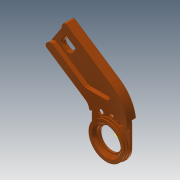
# Autodesk Inventor part: J009523
Saved by Autodesk Inventor 2020 (Build 240168000, 168)
## iProperties
RuleStatus: InUse
AfterDocSave0: file://Part Number Cleaner
Created: 2014-10-29
Material: TITANIUM, 6AL-4V, ANNEALED
Vendor: HHMI: JRC - JET
Document SubType Name: Modeling
Designer: arnoldj
Density: 4.43 g/cm^3
Description: MBS INLINE RING TAB THIN
Mass: 2.07661 g
Surface Area: 8.87594 cm^2
Volume: 0.468761 cm^3
Project: COMMON
Appearance: Smooth - Light Orange
Sheet Metal Rule: Default
Part Number: J009523
DESIGN DEPARTMENT: HHMI: JRC - ID&F
SPECIAL FINISH: NONE
LAB/DEPT: COMMON
REQUESTING SCIENTIST: COMMON
SURFACE ROUGHNESS: 63 Ra
Thickness: 0.100 in
ALTERED ITEM PART NUMBER: N/A
ALTERED ITEM VENDOR: N/A
ALTERED ITEM DESCRIPTION: N/A
Revision Number: -
Autodesk Inventor part; units mm, degrees
ref_plane "YZ Plane" through (0, 0, 0) normal (1, 0, 0) x (0, 1, 0)
sketch "Sketch1" plane through (0, 0, 0) normal (0, 0, 1) x (1, 0, 0)
  line L0 (-5.334, -5) -> (-5.334, 6.0312)
  line L1 (-5.334, 6.0312) -> (-5.334, -2.6352) construction
  line L2 (-5.334, 6.0312) -> (-17.9557, 14.3853)
  line L3 (-17.9557, 14.3853) -> (-12.4181, 22.7517)
  line L4 (-12.4181, 22.7517) -> (5.334, 11.0019)
  line L5 (-17.9557, 14.3853) -> (-30.248, 14.3853) construction
  line L6 (-15.1869, 18.5685) -> (0, 8.5166) construction
  line L7 (-12.1504, 14.2743) -> (-10.0476, 17.4514)
  line L8 (-10.0476, 17.4514) -> (-12.7163, 19.2178)
  line L9 (-12.7163, 19.2178) -> (-14.8192, 16.0407)
  line L10 (-14.8192, 16.0407) -> (-12.1504, 14.2743)
  line L11 (-12.1504, 14.2743) -> (-12.7163, 19.2178) construction
  line L12 (-10.0476, 17.4514) -> (-14.8192, 16.0407) construction
  circle A0 centre (0, 0) radius 3.5 construction
  line L13 (5.334, -5) -> (5.334, 11.0019)
  line L14 (0, 29.0086) -> (0, -14.7897) projected
  line L15 (-38.8526, 0) -> (21.3792, 0) projected
  circle A1 centre (0, 0) radius 3.5
  line L16 (-5.334, -5) -> (5.334, -5)
  point P0 (0, 0)
  point P1 (-2.611, 1.214)
  point P2 (-12.4334, 16.746)
  dimension "d161" = 123.5
  dimension "d162" = 10.033
  dimension "d177" = 146.5
  dimension "d221" = 3.302
  dimension "d232" = 3.2004
  dimension "d233" = 3.81
  dimension "d262" = 7
  dimension "d267" = 0
  dimension "d271" = 16.746
  dimension "d273" = 5.334
  dimension "d274" = 1.834
  dimension "d275" = 5.334
  dimension "d320" = 0
  dimension "d321" = 5
  dimension "d430" = 12.4334
  constraints: 30 end point, 4 coincident, 4 parallel, 4 point on line, 3 midpoint, 3 perpendicular, 3 vertical, 2 centre point, 2 horizontal, 1 concentric
  measures "d161" angle of L2 L0
  measures "d162" distance of L2.end L3.end
  measures "d177" angle of L2 L5
  measures "d221" distance from line of point (-12.433, 16.746) L3
  measures "d232" distance of L7.end L8.end
  measures "d233" distance of L7.start L7.end
  measures "d262" diameter of A0
  measures "d267" distance from line of L15 point (0, 0)
  measures "d271" vertical distance of point (-12.433, 16.746) A1.centre
  measures "d273" distance from line of A0.centre L0
  measures "d274" distance edge to line of A0 L0
  measures "d275" distance from line of A0.centre L13
  measures "d320" distance from line of L14 A0.centre
  measures "d321" distance from line of A0.centre L16
  measures "d430" distance from line of point (-12.433, 16.746) L14
extrude "Plate1" add sketch "Sketch1" along normal blind 2.54 contours L0 L15 A1 L14 L16 | L0 L2 L3 L4 L14 A1 L15 | L14 A1 L15 L13 L16 | L14 L4 L13 L15 A1 | L10 L9 L8 L7
ref_plane "Work Plane1" through (0, 10.16, 0) normal (0, 1, 0) x (-1, 0, 0)
sketch "Sketch7" plane through (0, 0, 0) normal (0, 0, 1) x (1, 0, 0)
  circle A0 centre (0, 6.0325) radius 0.8255
  circle A1 centre (-2.921, 5.1689) radius 0.8255
  circle A2 centre (2.921, 5.1689) radius 0.8255
  line L0 (0, 23.2371) -> (0, -13.8278) construction
  circle A3 centre (-2.1082, 6.9916) radius 0.8255
  circle A4 centre (2.1082, 6.9916) radius 0.8255
  line L1 (-5.334, -5) -> (-5.334, 6.0312) projected
  line L2 (-22.6717, 0) -> (18.6824, 0) projected
  circle A5 centre (0, 0) radius 3.5 projected
  circle A6 centre (0, 0) radius 6.0325 construction
  circle A7 centre (0, 0) radius 7.3025 construction
  dimension "d343" = 12.065
  dimension "d61" = 1.651
  dimension "d344" = 14.605
  dimension "d345" = 2.921
  dimension "d346" = 2.921
  dimension "d347" = 2.1082
  dimension "d348" = 2.1082
  constraints: 6 centre point, 5 coincident, 4 equal radius, 2 point on circle, 1 vertical alignment, 2 other
  measures "d61" diameter of A0
  measures "d344" diameter of A7
  measures "d345" horizontal distance of A0.centre point (2.921, 5.169)
  measures "d346" horizontal distance of point (-2.921, 5.169) A0.centre
  measures "d347" distance from line of L0 point (2.108, 6.992)
  measures "d348" distance from line of L0 A3.centre
hole "Hole2" at (-2.921, 5.1689, 0) at (2.921, 5.1689, 0) at (0, 6.0325, 0) direction (0, 0, 1) diameter 1.651 depth 2.54 tip angle 118
ref_plane "Work Plane3" through (0, 0, 1.143) normal (0, 0, 1) x (1, 0, 0)
sketch "Sketch9" plane through (0, 0, 0) normal (0, 0, 1) x (1, 0, 0)
  point P0 (0, 0)
sketch "Sketch10" plane through (0, 0, 0) normal (0, 0, 1) x (1, 0, 0)
  circle A0 centre (2.6461, -1.2506) radius 3.5
  point P0 (0, 0)
  dimension "d150" = 7
  constraints: 1 centre point
  measures "d150" diameter of A0
sketch "Sketch3" plane through (0, 0, 2.54) normal (0, 0, 1) x (1, 0, 0)
  line L0 (-16.764, 14.16) -> (4.445, 14.16)
  line L1 (-4.445, 6.16) -> (-16.764, 6.16)
  line L2 (-6.35, 14.16) -> (-6.35, 6.16)
  line L3 (0, 17.9421) -> (0, -8.5328)
  line L4 (12.7747, 8.2785) -> (4.445, 8.2785)
  point P0 (0, 0)
  point P1 (-5.2531, 14.0148)
  point P2 (4.445, 14.16)
  dimension "d15" = 6.35
  constraints: 8 end point, 1 perpendicular, 1 point on line, 4 other
  measures "d15" distance between parallel lines of L3 L2
sketch "Sketch15" plane through (0, 0, 0) normal (0, 0, 1) x (1, 0, 0)
  point P0 (0, 0)
extrude "Extrusion7" cut sketch "Sketch1" along normal up to next contours L10 L9 L8 L7
fillet "Fillet19" radius 1.27 4 edges at (-10.0476, 17.4514, 1.27) (-12.1504, 14.2743, 1.27) (-14.8192, 16.0407, 1.27) (-12.7163, 19.2178, 1.27)
sketch "Sketch20" plane through (0, 0, 2.54) normal (0, 0, 1) x (1, 0, 0)
  line L0 (-8.8901, 11.8492) -> (-7.334, 10.8192) projected
  arc A0 (-5.9889, 9.9289) -> (-5.2719, 9.9399) centre (-5.6384, 10.4584) ccw projected
  arc A1 (-1.4629, 11.8226) -> (-5.2719, 9.9399) centre (2.611, -1.214) ccw projected
  arc A2 (-1.4629, 11.8226) -> (-1.3018, 12.9582) centre (-1.6523, 12.4287) ccw projected
  line L1 (-0.9897, 12.7516) -> (-6.0681, 16.1129) projected
  line L2 (-17.9557, 14.3853) -> (-12.4181, 22.7517) projected
  line L3 (-3.6255, 8.3647) -> (-5.9889, 9.9289) projected
  point P0 (0, 0)
  point P1 (-6.15, 10.0356)
  point P2 (-14.4105, 15.5031)
  point P3 (-11.5885, 19.7667)
  point P4 (3.9211, 9.5012)
  point P5 (-4.6656, 9.0531)
  point P6 (2.0737, 10.7239)
  point P7 (-7.7842, 11.1172)
  point P8 (0.4848, 11.7756)
  point P9 (2.8447, 10.2136)
  point P10 (-5.8286, 9.8228)
  point P11 (-0.3868, 12.3525)
  constraints: 2 other
extrude "Extrusion11" [suppressed]
chamfer "Chamfer6" distance 0.254 angle 45 8 edges at (-10.563, 17.3465, 0) (-11.099, 15.8628, 0) (-12.2553, 14.7898, 0) (-13.4848, 15.1575, 0) (-14.3037, 16.1456, 0) (-13.7678, 17.6292, 0) (-12.6114, 18.7023, 0) (-11.3819, 18.3346, 0)
fillet "Fillet20" radius 0.635 2 edges at (-17.9557, 14.3853, 1.27) (-12.4181, 22.7517, 1.27)
ref_plane "Work Plane5" through (-12.7087, 16.9283, 0.254) normal (-0.551937, -0.8338858, 0) x (0.8338858, -0.551937, 0)
ref_plane "Work Plane6" through (-12.0829, 17.2755, 0.254) normal (-0.8338858, 0.551937, 0) x (0, 0, 1)
fillet "Fillet21" radius 2.54 1 edges at (-5.334, 6.0312, 1.27)
fillet "Fillet22" radius 5.08 2 edges at (-5.334, -5, 1.27) (5.334, -5, 1.27)
fillet "Fillet31" radius 10.16 1 edges at (5.334, 11.0019, 1.27)
sketch "Sketch25" plane through (0, 0, 0) normal (1, 0, 0) x (0, 1, 0)
  line L0 (1.27, 1.778) -> (4.064, 1.778)
  line L1 (5.08, 0.762) -> (5.08, 0)
  line L2 (-4.0321, 0) -> (13.299, 0)
  line L3 (5.08, 0) -> (1.27, 0)
  line L4 (1.27, 1.778) -> (1.27, 0)
  line L5 (0, -5.0635) -> (0, 5.7054) projected
  line L6 (1.27, 4.167) -> (1.27, -3.5251)
  arc A0 (5.08, 0.762) -> (4.064, 1.778) centre (4.064, 0.762) ccw
  line L7 (-5, 2.54) -> (0.08, 2.54) projected
  line L8 (-5, 2.54) -> (-5, 0) projected
  point P0 (5.08, 1.778)
  dimension "d324" = 2.54
  dimension "d325" = 0
  dimension "d326" = 3.81
  dimension "d327" = 1.016
  dimension "d328" = 0.762
  dimension "d352" = 6.27
  constraints: 12 end point, 3 point on line, 2 point on circle, 2 tangent, 2 vertical, 1 centre point, 1 perpendicular
  measures "d324" diameter of L5 L6
  measures "d325" distance between parallel lines of L4 L6
  measures "d326" distance of L0.start point (5.08, 1.778)
  measures "d327" radius of A0
  measures "d328" distance between parallel lines of L0 L7
  measures "d352" distance between parallel lines of L4 L8
sketch "Sketch26" plane through (0, 0, 2.54) normal (0, 0, 1) x (1, 0, 0)
  point P0 (0, 0)
sketch "Sketch27" plane through (0, 0, 2.54) normal (0, 0, 1) x (1, 0, 0)
  line L0 (-17.6052, 14.9149) -> (-12.7686, 22.2222) projected
  line L1 (-11.8886, 22.4012) -> (5.334, 11.0019) projected
  line L2 (-6.4721, 6.7845) -> (-17.4261, 14.0349) projected
  line L3 (-16.729, 16.2386) -> (-13.6448, 20.8984)
  line L4 (-13.6448, 20.8984) -> (-3.5839, 14.2393)
  line L5 (-3.5839, 14.2393) -> (-6.6681, 9.5795)
  line L6 (-6.6681, 9.5795) -> (-16.729, 16.2386)
  line L7 (-15.1869, 18.5685) -> (0, 8.5166) construction
  line L8 (-6.6681, 9.5795) -> (-0.7636, 9.5795)
  line L9 (-3.5839, 14.2393) -> (-0.0626, 11.9086)
  arc A0 (-0.7636, 9.5795) -> (-0.0626, 11.9086) centre (-0.7636, 10.8495) ccw
  point P0 (0, 0)
  point P1 (4.765, 11.3785)
  dimension "d334" = 12.065
  dimension "d335" = 5.588
  dimension "d429" = 2.2225
  dimension "d431" = 1.27
  constraints: 14 end point, 2 parallel, 2 point on circle, 2 point on line, 2 tangent, 1 centre point, 1 collinear, 1 horizontal, 1 midpoint, 1 perpendicular, 1 other
  measures "d334" distance of L3.end L4.end
  measures "d335" distance between parallel lines of L6 L4
  measures "d429" distance between parallel lines of L1 L4
  measures "d431" radius of A0
extrude "Extrusion13" cut sketch "Sketch27" against normal blind 1.27
fillet "Fillet26" radius 1.27 1 edges at (-6.6681, 9.5795, 1.905)
fillet "Fillet27" radius 1.27 2 edges at (-13.6448, 20.8984, 1.905) (-16.729, 16.2386, 1.905)
chamfer "Chamfer9" distance 0.254 angle 45 8 edges at (-12.6114, 18.7023, 1.27) (-13.7678, 17.6292, 1.27) (-14.3037, 16.1456, 1.27) (-13.4848, 15.1575, 1.27) (-12.2553, 14.7898, 1.27) (-11.099, 15.8628, 1.27) (-10.563, 17.3465, 1.27) (-11.3819, 18.3346, 1.27)
sketch "Sketch28" plane through (0, 0, 0) normal (0, 0, 1) x (1, 0, 0)
  line L0 (-4.1275, -5) -> (4.1275, -5)
  line L1 (4.1275, -5) -> (4.1275, 8.335)
  line L2 (4.1275, 8.335) -> (-4.1275, 8.335)
  line L3 (-4.1275, 8.335) -> (-4.1275, -5)
  line L4 (-4.1275, -5) -> (4.1275, 8.335) construction
  line L5 (4.1275, -5) -> (-4.1275, 8.335) construction
  line L6 (-0.254, -5) -> (0.254, -5) projected
  point P0 (0, 0)
  point P1 (0, 1.6675)
  dimension "d353" = 8.255
  dimension "d354" = 0
  dimension "d355" = 13.335
  constraints: 12 end point, 2 midpoint, 2 parallel, 1 horizontal, 1 perpendicular
  measures "d353" distance of L1.end L2.end
  measures "d354" distance from line of L6.start L0
  measures "d355" distance of L0.end L1.end
extrude "Extrusion14" cut sketch "Sketch28" along normal blind 1.27
fillet "Fillet28" radius 3.175 2 edges at (4.1275, 8.335, 0.635) (-4.1275, 8.335, 0.635)
chamfer "Chamfer10" distance 0.381 angle 45 5 edges at (4.1275, 0.9766, 0) (3.1976, 7.4051, 0) (0, 8.335, 0) (-3.1976, 7.4051, 0) (-4.1275, 0.9766, 0)
fillet "Fillet30" radius 0.381 2 edges at (4.1275, -3.2067, 0.8255) (-4.1275, -3.2067, 0.8255)
sketch "Sketch29" plane through (0, 0, 2.54) normal (0, 0, 1) x (1, 0, 0)
  point P0 (0, 0)
sketch "Sketch33" plane through (0, 0, 2.54) normal (0, 0, 1) x (1, 0, 0)
  circle A0 centre (0, 0) radius 3.5 projected
  circle A1 centre (0, 0) radius 3.5
  circle A2 centre (0, 0) radius 4.516 construction
  circle A3 centre (0, 0) radius 6.929
  circle A4 centre (0, 0) radius 5.024 construction
  circle A5 centre (-1.6762, 5.4715) radius 1.2065 construction
  circle A6 centre (-1.6762, 5.4715) radius 0.5969 construction
  dimension "d383" = 1.016
  dimension "d384" = 2.413
  dimension "d395" = 0.508
  dimension "d396" = 2.413
  dimension "d397" = 1.1938
  constraints: 6 centre point, 5 coincident, 2 tangent, 1 concentric
  measures "d383" radial gap between concentric circles of A2 A0
  measures "d384" radial gap between concentric circles of A2 A3
  measures "d395" radial gap between concentric circles of A2 A4
  measures "d396" diameter of A5
  measures "d397" diameter of A6
extrude "Extrusion17" cut sketch "Sketch33" against normal blind 0.762 contours A0 | A3
sketch "Sketch37" plane through (0, 0, 1.778) normal (0, 0, 1) x (1, 0, 0)
  circle A0 centre (0, 0) radius 3.5 projected
  circle A1 centre (0, 0) radius 3.5
  circle A2 centre (0, 0) radius 4.5668
  dimension "d419" = 1.0668
  constraints: 2 centre point, 1 coincident, 1 concentric
  measures "d419" radial gap between concentric circles of A0 A2
extrude "Extrusion21" add sketch "Sketch37" along normal blind 0.889
fillet "Fillet32" radius 0.254 2 edges at (-5.334, 4.4226, 2.159) (5.334, 4.4226, 2.159)
hole "Hole4" at (0, 0, 1.27) direction (0, 0, 1) diameter 8 depth 0.1524
sketch "Sketch23" plane through (0, 0, 0) normal (0, 0, -1) x (-1, 0, 0)
  line L0 (-5.334, 11.0019) -> (11.8886, 22.4012) projected
  line L1 (12.7686, 22.2222) -> (17.6052, 14.9149) projected
  line L2 (17.4261, 14.0349) -> (6.4721, 6.7845) projected
  line L3 (12.3803, 22.7267) -> (17.9179, 14.3604)
  line L4 (17.9179, 14.3604) -> (10.2882, 9.3104)
  line L5 (10.2882, 9.3104) -> (4.7507, 17.6768)
  line L6 (4.7507, 17.6768) -> (12.3803, 22.7267)
  line L7 (17.6052, 14.9149) -> (12.7686, 22.2222) projected
  point P0 (0, 0)
  point P1 (-4.765, 11.3785)
  dimension "d316" = 9.1948
  constraints: 8 end point, 3 parallel, 1 perpendicular
  measures "d316" distance between parallel lines of L1 L5
feature "Simulation Only Cut4" [suppressed]
sketch "Sketch16" plane through (0, 0, 0) normal (0, 0, 1) x (1, 0, 0)
  circle A0 centre (0, 3.349) radius 0.1979
  circle A1 centre (0, 0) radius 3.5 projected
  constraints: 1 centre point, 1 vertical alignment
extrude "Simulation Only Extrusion8" [suppressed]
sketch "Sketch35" plane through (0, 0, 1.4224) normal (0, 0, -1) x (-1, 0, 0)
  circle A0 centre (0, 0) radius 3.5 projected
  circle A1 centre (0, 0) radius 4 projected
  circle A2 centre (0, 0) radius 4 projected
  circle A3 centre (0, 0) radius 3.119
  dimension "d409" = 0.381
  constraints: 1 centre point
  measures "d409" radial gap between concentric circles of A0 A3
extrude "Extrusion19" add sketch "Sketch35" against normal blind 0.508 contours A0
sketch "Sketch36" plane through (0, 0, 1.778) normal (0, 0, 1) x (1, 0, 0)
  circle A0 centre (0, 0) radius 4.516 projected
  circle A1 centre (0, 0) radius 5.024 projected
extrude "Extrusion20" add sketch "Sketch36" along normal blind 0.381
sketch "Sketch38" plane through (0, 0, 2.667) normal (0, 0, 1) x (1, 0, 0)
  circle A0 centre (0, 0) radius 5.024 projected
  circle A1 centre (0, 0) radius 3.5 projected
extrude "Extrusion22" add sketch "Sketch38" along normal blind 0.381
chamfer "Chamfer13" distance 0.635 angle 45 1 edges at (-3.5, 0, 3.048)
sketch "Sketch39" plane through (0, 0, 0) normal (0, 0, -1) x (-1, 0, 0)
  point P0 (0, 0)
sketch "Sketch40" plane through (0, 0, 0) normal (0, 0, -1) x (-1, 0, 0)
  arc A0 (4.5085, -2.296) -> (4.8535, -2.0767) centre (4.5085, -1.915) ccw projected
  arc A1 (4.8535, -2.0767) -> (5.334, 0.08) centre (0.254, 0.08) ccw projected
  line L0 (5.334, 4.6665) -> (5.334, 0.08) projected
  arc A2 (6.4721, 6.7845) -> (5.334, 4.6665) centre (7.874, 4.6665) ccw projected
  line L1 (17.4261, 14.0349) -> (6.4721, 6.7845) projected
  arc A3 (17.4261, 14.0349) -> (17.6052, 14.9149) centre (17.0757, 14.5644) ccw projected
  line L2 (12.7686, 22.2222) -> (17.6052, 14.9149) projected
  arc A4 (12.7686, 22.2222) -> (11.8886, 22.4012) centre (12.239, 21.8717) ccw projected
  line L3 (-0.7817, 14.015) -> (11.8886, 22.4012) projected
  arc A5 (-0.7817, 14.015) -> (-5.334, 5.5427) centre (4.826, 5.5427) ccw projected
  line L4 (-5.334, 0.08) -> (-5.334, 5.5427) projected
  arc A6 (-5.334, 0.08) -> (-4.8535, -2.0767) centre (-0.254, 0.08) ccw projected
  arc A7 (-4.8535, -2.0767) -> (-4.5085, -2.296) centre (-4.5085, -1.915) ccw projected
  line L5 (-4.5085, 5.16) -> (-4.5085, -2.296) projected
  arc A8 (-0.9525, 8.716) -> (-4.5085, 5.16) centre (-0.9525, 5.16) ccw projected
  line L6 (0.9525, 8.716) -> (-0.9525, 8.716) projected
  arc A9 (4.5085, 5.16) -> (0.9525, 8.716) centre (0.9525, 5.16) ccw projected
  line L7 (4.5085, -2.296) -> (4.5085, 5.16) projected
  arc A10 (10.9664, 18.3641) -> (10.5367, 16.2521) centre (11.8075, 17.0933) ccw projected
  line L8 (11.5171, 18.7286) -> (10.9664, 18.3641) projected
  arc A11 (13.6291, 18.2989) -> (11.5171, 18.7286) centre (12.3582, 17.4578) ccw projected
  line L9 (14.33, 17.2399) -> (13.6291, 18.2989) projected
  arc A12 (13.9004, 15.1279) -> (14.33, 17.2399) centre (13.0592, 16.3988) ccw projected
  line L10 (13.3497, 14.7634) -> (13.9004, 15.1279) projected
  arc A13 (11.2377, 15.1931) -> (13.3497, 14.7634) centre (12.5085, 16.0343) ccw projected
  line L11 (10.5367, 16.2521) -> (11.2377, 15.1931) projected
  line L12 (0, -14.756) -> (0, 28.8067) projected
  line L13 (-18.8871, 0) -> (23.8999, 0) projected
  line L14 (-7.62, 6.858) -> (7.62, 6.858)
  line L15 (7.62, 6.858) -> (7.62, -5.842)
  line L16 (7.62, -5.842) -> (-7.62, -5.842)
  line L17 (-7.62, -5.842) -> (-7.62, 6.858)
  line L18 (-7.62, 6.858) -> (7.62, -5.842) construction
  line L19 (7.62, 6.858) -> (-7.62, -5.842) construction
  circle A14 centre (0, 6.0325) radius 0.8255 projected
  point P0 (0, 0)
  point P1 (0, 0.508)
  dimension "d433" = 12.7
  dimension "d434" = 15.24
  constraints: 12 end point, 2 midpoint, 2 parallel, 1 horizontal, 1 perpendicular, 1 point on line, 1 tangent
  measures "d433" distance of L14.end L15.end
  measures "d434" distance of L15.end L16.end
extrude "Extrusion23" cut sketch "Sketch40" against normal blind 1.143 contours L7 L13 A1 A0 | A0 A1 L13 L15 L16 L12 L7 | L13 L12 A14 L14 A9 L7 | L7 A9 L14 L1 A2 L0 A1 L13 | A1 L0 A2 L1 L14 L15 L13 | L13 L5 A8 L14 A14 L12 | L12 L16 L17 L13 A6 A7 L5 | A14 L12 | L12 A14 | L13 A6 L4 A5 L14 A8 L5 | L5 A7 A6 L13 | L13 L17 L14 A5 L4 A6
equation "\"d71\" = Thickness"
equation "\"BendRadius\" = Thickness"
equation "\"BendReliefWidth\" = Thickness"
equation "\"BendReliefDepth\" = 0.5 * Thickness"
equation "\"CornerReliefSize\" = 4 * Thickness"
equation "\"MinimumRemnant\" = 2 * Thickness"
equation "\"TransitionRadius\" = BendRadius"
equation "\"JacobiRadiusSize\" = BendRadius"
equation "\"GapSize\" = Thickness"
equation "\"d6\" = BendRadius"
equation "\"Thickness\" = 2.54"
body "Solid1"
